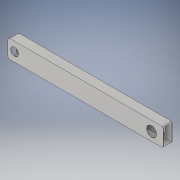
# Autodesk Inventor part: SideBar15
Saved by Autodesk Inventor 2018.3 (Build 223284000, 284)
## iProperties
Created: 2020-01-25
Part Number: SideBar15
Material: Aluminum 6061
Document SubType Name: Modeling
Designer: Myers
Mass: 261.234 g
Surface Area: 1229.33 cm^2
Volume: 96.7533 cm^3
Density: 2.7 g/cm^3
Appearance: Aluminum - Dark
Author: Myers
Autodesk Inventor part; units mm, degrees
ref_plane "YZ Plane" through (0, 0, 0) normal (1, 0, 0) x (0, 1, 0)
ref_plane "XZ Plane" through (0, 0, 0) normal (0, 1, 0) x (-1, 0, 0)
ref_plane "XY Plane" through (0, 0, 0) normal (0, 0, 1) x (1, 0, 0)
sketch "Sketch1" plane through (0, 0, 0) normal (0, 0, 1) x (1, 0, 0)
  line L0 (-211.1358, -25.4) -> (211.1358, -25.4)
  line L1 (214.3108, -22.225) -> (214.3108, 22.225)
  line L2 (211.1358, 25.4) -> (-211.1358, 25.4)
  line L3 (-217.4858, 19.05) -> (-217.4858, -19.05)
  circle A0 centre (-198.4358, 0) radius 11.1125
  circle A1 centre (182.5608, -1.5875) radius 14.2875
  arc A2 (-217.4858, -19.05) -> (-211.1358, -25.4) centre (-211.1358, -19.05) ccw
  arc A3 (-211.1358, 25.4) -> (-217.4858, 19.05) centre (-211.1358, 19.05) ccw
  arc A4 (214.3108, 22.225) -> (211.1358, 25.4) centre (211.1358, 22.225) ccw
  arc A5 (211.1358, -25.4) -> (214.3108, -22.225) centre (211.1358, -22.225) ccw
  point P0 (0, 0)
  point P1 (-217.4858, -25.4)
  point P2 (214.3108, 25.4)
  point P3 (214.3108, -25.4)
  point P4 (-217.4858, 25.4)
  point P5 (-217.4858, 0)
  point P6 (0, 25.4)
  point P7 (214.3108, -19.05)
  point P8 (200.025, -25.4)
  point P9 (214.3108, 6.35)
  point P10 (195.2625, 25.4)
  dimension "d6" = 22.225
  dimension "d8" = 19.05
  dimension "d9" = 50.8
  dimension "d11" = 6.35
  dimension "d15" = 31.75
  dimension "d16" = 3.175
  dimension "d17" = 28.575
  dimension "d18" = 23.8125
  dimension "d19" = 380.9967
  constraints: 12 point on line, 8 end point, 8 point on circle, 8 tangent, 6 centre point, 2 equal radius, 2 horizontal alignment, 2 midpoint, 2 parallel, 1 horizontal, 1 perpendicular, 1 vertical alignment
  measures "d6" diameter of A0
  measures "d8" distance from line of A0.centre L3
  measures "d9" distance of point (214.311, -25.4) point (214.311, 25.4)
  measures "d11" radius of A3
  measures "d15" distance from line of L1 A1.centre
  measures "d16" radius of A4
  measures "d17" diameter of A1
  measures "d18" distance from line of L0 A1.centre
  measures "d19" horizontal distance of A0.centre A1.centre
extrude "Extrusion1" add sketch "Sketch1" along normal blind 25.4
sketch "Sketch2" plane through (0, 0, 0) normal (1, 0, 0) x (0, 1, 0)
  line L0 (25.4, 0) -> (25.4, 25.4) projected
  line L1 (25.4, 25.4) -> (19.05, 25.4) projected
  line L2 (19.05, 25.4) -> (-19.05, 25.4) projected
  line L3 (-19.05, 25.4) -> (-25.4, 25.4) projected
  line L4 (-25.4, 0) -> (-25.4, 25.4) projected
  line L5 (-19.05, 0) -> (-25.4, 0) projected
  line L6 (19.05, 0) -> (-19.05, 0) projected
  line L7 (25.4, 0) -> (19.05, 0) projected
  line L8 (23.8125, 23.8125) -> (23.8125, 1.5875)
  line L9 (23.8125, 1.5875) -> (12.7, 1.5875)
  line L10 (12.7, 1.5875) -> (-12.7, 1.5875)
  line L11 (-12.7, 1.5875) -> (-23.8125, 1.5875)
  line L12 (-23.8125, 1.5875) -> (-23.8125, 23.8125)
  line L13 (-23.8125, 23.8125) -> (-12.7, 23.8125)
  line L14 (-12.7, 23.8125) -> (12.7, 23.8125)
  line L15 (12.7, 23.8125) -> (23.8125, 23.8125)
  point P0 (0, 0)
  dimension "d12" = 1.5875
  constraints: 16 end point, 7 other
  measures "d12" distance between parallel lines of L0 L8
extrude "Extrusion2" cut sketch "Sketch2" along normal through all both and the other way through all contours L8 L9 L10 L11 L12 L13 L14 L15
body "Solid1"
